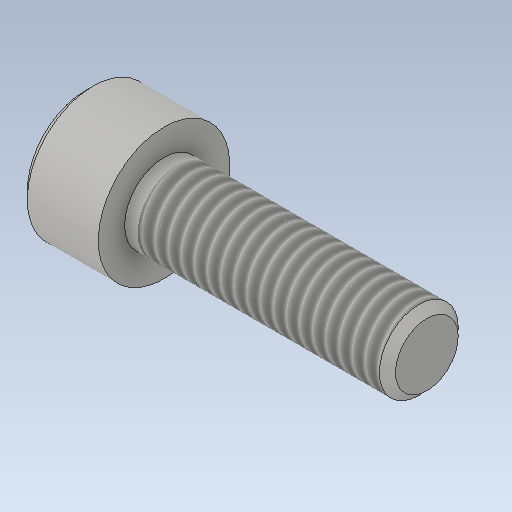
# Autodesk Inventor part: BOLT6-20
Saved by Autodesk Inventor 2020.2 (Build 242310000, 310)
## iProperties
Created: 2022-11-16
Part Number: BOLT6-20
Material: Generic
Catalog Web Link: www.cadenas.de
Description: BOLT-Hexagon Socket Head Cap Screws
Vendor: MISUMI
Document SubType Name: Modeling
Designer: psAdmin
Manufacturer: MISUMI
Mass: 0.958655 g
Surface Area: 7.56446 cm^2
Volume: 0.958655 cm^3
Density: 1 g/cm^3
Appearance: PSOLRGB-175-175-175
Category: PARTsolutions
Company: MISUMI
PSOL_IDENT_0: {$CADENAS_DATA/23d-libs/misumi/metric/accessories/bolt.prj},157 {VTYP=3D},{NB=BOLT6-20},{LINA=BOLT6-
PSOL_IDENT_1: 20},{NN=BOLT},{DATE=30.06.2021 13:30:08},{GEOMDATE=12.05.2017 08:21:09},{VERSION=},{LINEID=120},{WBV
PSOL_IDENT_2: AR=L},{WBNUMERIC=L}  {NB=BOLT6-20},{LINA=BOLT6-20},{KT=DUMMY},{PN=BOLT6-20},{TYPE=BOLT},{L=20.0},{M=
PSOL_IDENT_3: 6.0},{P=1},{A=10.0},{E=6.0},{B=5.0},{C=0.60},{LL=0}
NB: BOLT6-20
NN: BOLT
NT: Hexagon Socket Head Cap Screws
NBSYN: $PN.
LINA: BOLT6-20
CATALOG: Misumi
PN: BOLT6-20
L: 20
M: 6
P: 1
C: 0.6
SUPPLIER: MISUMI
ARTICLENO: BOLT6-20
BOMINFO: BOLT6-20
CREATOR: CADENAS GmbH
Title: BOLT6-20
Author: Cadenas PARTsolutions
Comments: Hexagon Socket Head Cap Screws
Autodesk Inventor part; units mm, degrees
sketch "Sketch_1" plane through (0, 0, 0) normal (0, 0, 1) x (1, 0, 0)
  line L0 (20, 0) -> (-6, 0)
  line L1 (-6, 0) -> (-6, 4.4)
  line L2 (-6, 4.4) -> (-5.4, 5)
  line L3 (-5.4, 5) -> (0, 5)
  line L4 (0, 5) -> (0, 3)
  line L5 (0, 3) -> (19.3865, 3)
  line L6 (19.3865, 3) -> (20, 2.3865)
  line L7 (20, 2.3865) -> (20, 0)
  line L8 (20, 0) -> (-6, 0)
  constraints: 18 end point
revolve "Revolution1" add sketch "Sketch_1" angle 360 about axis through (20, 0, 0) along (1, 0, 0)
thread "Thread1" size "M6x1" class "6g" standard "ISO Metric profile" length 18.3865
sketch "Sketch2" plane through (-6, 0, 0) normal (-1, 0, 0) x (0, 0, 1)
  point P0 (0, 0)
hole "Hole1" at (-6, 0, 0) direction (1, 0, 0) diameter 5 depth 3 tip angle 150
sketch "Sketch_3" plane through (-6, 0, 0) normal (1, 0, 0) x (0, 0, -1)
  line L0 (-2.5, -1.4434) -> (0, -2.8868)
  line L1 (0, -2.8868) -> (2.5, -1.4434)
  line L2 (2.5, -1.4434) -> (2.5, 1.4434)
  line L3 (2.5, 1.4434) -> (0, 2.8868)
  line L4 (0, 2.8868) -> (-2.5, 1.4434)
  line L5 (-2.5, 1.4434) -> (-2.5, -1.4434)
  constraints: 12 end point
extrude "Extrusion1" cut sketch "Sketch_3" along normal blind 3
ref_plane "to_cp_XY" through (0, 0, 0) normal (1, 0, 0) x (0, 0, -1)
ref_plane "to_cp_YZ" through (0, 0, 0) normal (0, 0, -1) x (0, 1, 0)
ref_plane "to_cp_ZX" through (0, 0, 0) normal (0, 1, 0) x (1, 0, 0)
body "Solid1"
